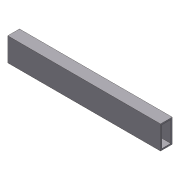
# Autodesk Inventor part: Frame_MainShooterFrame_FrontRear
Saved by Autodesk Inventor 2012 (Build 160160000, 160)
## iProperties
Created: 2012-01-21
Part Number: Frame_MainShooterFrame_FrontRear
Material: Aluminum-6061
Document SubType Name: Modeling
Designer: JesseK
Mass: 396.905 g
Surface Area: 931.45 cm^2
Volume: 146.459 cm^3
Density: 2.71 g/cm^3
Author: JesseK
Autodesk Inventor part; units mm, degrees
ref_plane "YZ Plane" through (0, 0, 0) normal (1, 0, 0) x (0, 1, 0)
ref_plane "XZ Plane" through (0, 0, 0) normal (0, 1, 0) x (-1, 0, 0)
ref_plane "XY Plane" through (0, 0, 0) normal (0, 0, 1) x (1, 0, 0)
sketch "Sketch1" plane through (0, 0, 0) normal (0, 0, 1) x (1, 0, 0)
  line L0 (0, 0) -> (330.2, 0)
  line L1 (330.2, 0) -> (330.2, 50.8)
  line L2 (330.2, 50.8) -> (0, 50.8)
  line L3 (0, 50.8) -> (0, 0)
  dimension "d0" = 330.2
  dimension "d1" = 50.8
  constraints: 8 end point, 2 parallel, 1 horizontal, 1 perpendicular
  measures "d0" distance of L1.end L2.end
  measures "d1" distance of L2.end L0.start
extrude "Extrusion1" add sketch "Sketch1" along normal blind 25.4
shell "Shell1" thickness 3.175 removed faces 2 at (0, 33.8667, 16.9333) at (330.2, 16.9333, 8.4667)
body "Solid1"
